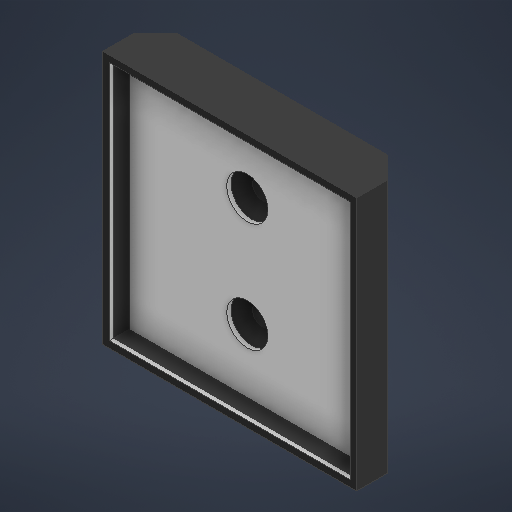
# Autodesk Inventor part: Werkstückträger
Saved by Autodesk Inventor 2026.1 (Build 301233020, 233B)
## iProperties
Created: 2024-12-08
Part Number: Werkstückträger
Material: Generisch
Document SubType Name: Modeling
Designer: florian.eder
Density: 1 g/cm^3
Appearance: Vorgabe
Author: florian.eder
Autodesk Inventor part; units mm, degrees
ref_plane "YZ Plane" through (0, 0, 0) normal (1, 0, 0) x (0, 1, 0)
ref_plane "XZ Plane" through (0, 0, 0) normal (0, 1, 0) x (-1, 0, 0)
ref_plane "XY Plane" through (0, 0, 0) normal (0, 0, 1) x (1, 0, 0)
sketch "Skizze1" plane through (0, 0, 0) normal (0, 1, 0) x (-1, 0, 0)
  line L0 (29, 29) -> (-29, 29)
  line L1 (-29, 29) -> (-29, -29)
  line L2 (-29, -29) -> (29, -29)
  line L3 (29, -29) -> (29, 29)
  line L4 (29, 29) -> (-29, -29) construction
  line L5 (-29, 29) -> (29, -29) construction
  line L6 (27, -27) -> (-27, -27)
  line L7 (-27, -27) -> (-27, 27)
  line L8 (-27, 27) -> (27, 27)
  line L9 (32.5, 0) -> (-32.5, 0)
  line L10 (27, 27) -> (-27, 27)
  line L11 (-27, 27) -> (-27, -27)
  line L12 (-27, -27) -> (27, -27)
  line L13 (27, 27) -> (27, -27)
  line L14 (27, 27) -> (27, -27)
  point P0 (0, 0)
  point P1 (-27, 0)
  point P2 (-210, -122)
  point P3 (0, 0)
  point P4 (29, 0)
  dimension "d0" = 58
  dimension "d1" = 58
  dimension "d5" = 2
  dimension "d8" = 54
  dimension "d9" = 2
  dimension "d10" = 56
  constraints: 30 end point, 6 midpoint, 4 symmetric about line, 3 equal length, 3 horizontal, 3 perpendicular, 1 vertical, 1 vertical alignment
  measures "d0" distance between parallel lines of L1 L3
  measures "d1" distance between parallel lines of L0 L2
  measures "d5" distance from line of L3 L8.end
  measures "d8" distance between parallel lines of L8 L6
  measures "d9" distance between parallel lines of L2 L6
  measures "d10" distance from line of point (-27, 0) L3
extrude "Extrusion1" add sketch "Skizze1" along normal blind 10
chamfer "Fasen3" distance 5 angle 45 1 edges at (29, 10, 0)
chamfer "Fasen4" distance 5 angle 45 1 edges at (-29, 10, 0)
extrude "Extrusion7" cut sketch "Skizze1" along normal blind 3 contours L13 L6 L7 L9 | L9 L7 L8 L13
sketch "Skizze7" plane through (0, 3, 0) normal (0, -1, 0) x (1, 0, 0)
  point P0 (0, 0)
  point P1 (0, 12.5)
  point P2 (0, -12.5)
  dimension "d76" = 25
  dimension "d77" = 12.5
  constraints: 2 vertical alignment
  measures "d76" distance of point (0, -12.5) point (0, 12.5)
  measures "d77" distance of point (0, 0) point (0, -12.5)
hole "Bohrung4" at (0, 3, 12.5) at (0, 3, -12.5) direction (0, 1, 0) diameter 4.5 end through all countersink diameter 9.4 countersink angle 90 clearance for "Flachkopfmaschinenschraube" size "M4" standard "ANSI Metrisches M Profil"
sketch "Skizze8" plane through (0, 10, 0) normal (0, 1, 0) x (1, 0, 0)
  circle A0 centre (0, 12.5) radius 2.25 projected
  circle A1 centre (0, 12.5) radius 3.05
  circle A2 centre (0, -12.5) radius 2.25 projected
  circle A3 centre (0, -12.5) radius 3.05
  point P0 (0, 0)
  dimension "d85" = 6.1
  dimension "d86" = 6.1
  constraints: 2 centre point, 2 coincident
  measures "d85" diameter of A1
  measures "d86" diameter of A3
extrude "Extrusion8" cut sketch "Skizze8" against normal blind 3.1
sketch "Skizze9" plane through (29, 0, -29) normal (0, 0, -1) x (-1, 0, 0)
  line L0 (0, 0) -> (0, 5) projected
  line L1 (29, 0) -> (29, 10)
  line L2 (53, 10) -> (5, 10) projected
  line L3 (56, 3) -> (2, 3) projected
  circle A0 centre (10, 6.5) radius 3
  point P0 (29, 5)
  dimension "d96" = 6
  dimension "d97" = 3.5
  dimension "d98" = 10
  constraints: 2 end point, 2 midpoint, 1 centre point
  measures "d96" diameter of A0
  measures "d97" distance from line of L2 A0.centre
  measures "d98" distance from line of L0 A0.centre
extrude "Extrusion9" cut sketch "Skizze9" against normal blind 3
sketch "Sketch11" plane through (0, 3, 0) normal (0, -1, 0) x (1, 0, 0)
  circle A0 centre (0, -12.5) radius 4.7 projected
  circle A1 centre (0, 12.5) radius 4.7 projected
  line L0 (-27, 27) -> (27, 27) projected
  line L1 (-27, -27) -> (-27, 27) projected
  line L2 (27, -27) -> (-27, -27) projected
  line L3 (27, 27) -> (27, -27) projected
  point P0 (0, 0)
extrude "Extrusion11" add sketch "Sketch11" along normal blind 1
thicken "Verdickung1" operation add thickness 2 both sides no extend neighbours no toward (0, -1, 0) faces at (-9, 0, -28.3333)
chamfer "Fasen5" distance 0.5 angle 45 1 edges at (27, -2, 0)
chamfer "Fasen6" distance 0.5 angle 45 5 edges at (27.25, -2, 27) (0, -2, 27) (-27, -2, 0) (27.25, -2, -27) (0, -2, -27)
equation "\"d77\" = 0.5 * d76"
